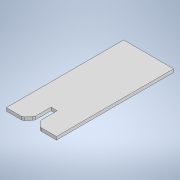
# Autodesk Inventor part: avbay sled
Saved by Autodesk Inventor 2020 (Build 240168000, 168)
## iProperties
Created: 2020-10-12
Part Number: avbay sled
Material: Generic
Document SubType Name: Modeling
Designer: mulve
Density: 1 g/cm^3
Appearance: Default
Author: mulve
Autodesk Inventor part; units mm, degrees
ref_plane "YZ Plane" through (0, 0, 0) normal (1, 0, 0) x (0, 1, 0)
ref_plane "XZ Plane" through (0, 0, 0) normal (0, 1, 0) x (-1, 0, 0)
ref_plane "XY Plane" through (0, 0, 0) normal (0, 0, 1) x (1, 0, 0)
sketch "Sketch1" plane through (0, 0, 0) normal (0, 1, 0) x (-1, 0, 0)
  line L0 (0, 0) -> (48.3455, 0)
  line L1 (48.3455, 0) -> (48.3455, -113.25)
  line L2 (48.3455, -113.25) -> (0, -113.25)
  line L3 (0, -113.25) -> (0, 0)
  line L4 (27.1728, 0) -> (21.1727, 0)
  line L5 (21.1727, 0) -> (21.1727, -21.95)
  line L6 (21.1727, -21.95) -> (27.1728, -21.95)
  line L7 (27.1728, -21.95) -> (27.1728, 0)
  line L8 (29.1728, 0) -> (19.1728, 0)
  line L9 (19.1728, 0) -> (19.1728, -3.302)
  line L10 (19.1728, -3.302) -> (29.1728, -3.302)
  line L11 (29.1728, -3.302) -> (29.1728, 0)
  point P0 (27.1728, -3.302)
  point P1 (21.1727, -3.302)
  dimension "d0" = 113.25
  dimension "d1" = 48.3455
  dimension "d2" = 91.3
  dimension "d3" = 6
  dimension "d4" = 21.1728
  dimension "d5" = 21.1728
  dimension "d6" = 10
  dimension "d7" = 3.302
  dimension "d8" = 2
  dimension "d9" = 2
  constraints: 24 end point, 6 parallel, 3 horizontal, 3 perpendicular, 2 point on line
  measures "d0" distance of L0.end L1.end
  measures "d1" distance of L0.start L0.end
  measures "d2" distance between parallel lines of L2 L6
  measures "d3" distance between parallel lines of L5 L7
  measures "d4" distance between parallel lines of L1 L7
  measures "d5" distance between parallel lines of L3 L5
  measures "d6" distance of L9.end L10.end
  measures "d7" distance between parallel lines of L10 L0
  measures "d8" distance between parallel lines of L5 L9
  measures "d9" distance between parallel lines of L7 L11
extrude "Extrusion1" add sketch "Sketch1" along normal mid plane 3 contours L0 L9 L10 L5 L6 L7 L11 L1 L2 L3
sketch "Sketch2" plane through (0, 1.5, 0) normal (0, 1, 0) x (1, 0, 0)
  line L0 (-48.3455, 0) -> (-29.1728, 0) projected
  line L1 (-32.4278, 0) -> (-15.9178, 0)
  line L2 (-15.9178, 0) -> (-24.1728, 9.721)
  line L3 (-24.1728, 9.721) -> (-32.4278, 0)
  line L4 (-29.1728, 0) -> (-29.1728, 3.302) projected
  line L5 (-19.1728, 3.302) -> (-19.1728, 0) projected
  point P0 (0, 0)
  dimension "d12" = 8.255
  dimension "d13" = 16.51
  dimension "d14" = 8.255
  dimension "d15" = 3.255
  dimension "d16" = 3.255
  constraints: 6 end point, 1 collinear, 1 point on line
  measures "d12" horizontal distance of L1.start L2.end
  measures "d13" distance of L1.start L1.end
  measures "d14" horizontal distance of L2.end L1.end
  measures "d15" distance from line of L4 L1.start
  measures "d16" distance from line of L5 L1.end
extrude "Extrusion2" cut sketch "Sketch2" against normal up to surface (3 mm away)
fillet "Fillet1" radius 3.175 4 edges at (-27.1728, 0, -6.1882) (-21.1728, 0, -6.1882) (-32.4278, 0, 0) (-15.9178, 0, 0)
equation "\"d4\" = d5"
equation "\"d8\" = d9"
equation "\"d12\" = d14"
equation "\"d15\" = d16"
body "Solid1"
